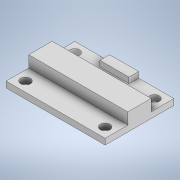
# Autodesk Inventor part: IMU-mpu6050
Saved by Autodesk Inventor 2022 (Build 260153000, 153)
## iProperties
Created: 2021-10-21
Part Number: IMU-mpu6050
Material: Generic
Document SubType Name: Modeling
Designer: kylem
Density: 1 g/cm^3
Appearance: Default
Author: kylem
Autodesk Inventor part; units mm, degrees
ref_plane "YZ Plane" through (0, 0, 0) normal (1, 0, 0) x (0, 1, 0)
ref_plane "XZ Plane" through (0, 0, 0) normal (0, 1, 0) x (-1, 0, 0)
sketch "Sketch1" plane through (0, 0, 0) normal (0, 1, 0) x (-1, 0, 0)
  line L0 (0, 0) -> (25.5, 0)
  line L1 (25.5, 0) -> (25.5, -17.7)
  line L2 (25.5, -17.7) -> (0, -17.7)
  line L3 (0, -17.7) -> (0, 0)
  dimension "d0" = 25.5
  dimension "d1" = 17.7
  constraints: 8 end point, 2 parallel, 1 horizontal, 1 perpendicular
  measures "d0" distance of L1.end L2.end
  measures "d1" distance of L0.end L1.end
extrude "Extrusion1" add sketch "Sketch1" along normal blind 1.54
sketch "Sketch2" plane through (0, 1.54, 0) normal (0, 1, 0) x (1, 0, 0)
  line L0 (-25.5, 0) -> (0, 0) projected
  line L1 (0, 0) -> (-2.5, 0)
  line L2 (-2.5, 0) -> (-2.5, 1.25)
  line L3 (-2.5, 2.5) -> (0, 2.5)
  line L4 (0, 2.5) -> (0, 0)
  circle A0 centre (-2.5, 2.5) radius 1.25
  line L5 (0, 17.7) -> (-25.5, 17.7) projected
  line L6 (0, 0) -> (0, 17.7)
  line L7 (0, 17.7) -> (0, 8.85)
  line L8 (0, 0) -> (0, 17.7) projected
  line L9 (0, 8.85) -> (-1.25, 8.85)
  line L10 (-25.5, 17.7) -> (0, 17.7)
  line L11 (-12.75, 17.7) -> (-12.75, 15.5963)
  circle A1 centre (-23, 2.5) radius 1.25
  circle A2 centre (-2.5, 15.2) radius 1.25
  circle A3 centre (-23, 15.2) radius 1.25
  dimension "d6" = 2.5
  dimension "d4" = 2.5
  dimension "d5" = 2.5
  constraints: 18 end point, 3 centre point, 3 symmetric about line, 2 horizontal, 2 midpoint, 2 parallel, 2 vertical, 1 coincident, 1 collinear, 1 perpendicular, 1 vertical alignment, 5 other
  measures "d4" distance of L3.start L3.end
  measures "d5" distance of L1.end L3.start
extrude "Extrusion2" cut sketch "Sketch2" against normal blind 1.54 contours A0 | A1 | A2 | A3
sketch "Sketch3" plane through (0, 0, 0) normal (1, 0, 0) x (0, 0, -1)
  line L0 (0, 0) -> (0, 1.54) projected
  line L1 (17.7, 0) -> (17.7, 1.54) projected
  line L2 (0, 0) -> (17.7, 0)
  line L3 (0, 0) -> (17.7, 0) projected
  line L4 (8.85, 0) -> (11.85, 0)
  line L5 (11.85, 0) -> (11.85, 4.5)
  line L6 (11.85, 4.5) -> (5.85, 4.5)
  line L7 (5.85, 4.5) -> (5.85, 0)
  line L8 (5.85, 4.5) -> (11.85, 4.5)
  line L9 (11.85, 4.5) -> (11.85, 0)
  line L10 (11.85, 0) -> (5.85, 0)
  line L11 (5.85, 0) -> (5.85, 4.5)
  dimension "d9" = 3
  dimension "d10" = 4.5
  dimension "d11" = 6
  constraints: 18 end point, 4 perpendicular, 2 horizontal, 2 parallel, 2 point on line, 1 midpoint
  measures "d9" distance of L4.start L4.end
  measures "d10" distance of L4.end L5.end
  measures "d11" distance of L5.end L6.end
extrude "Extrusion3" add sketch "Sketch3" against normal blind 25.5
sketch "Sketch4" plane through (0, 0, 0) normal (0, -1, 0) x (1, 0, 0)
  line L0 (0, -17.7) -> (-25.5, -17.7) projected
  line L1 (-9.0744, -17.7) -> (-16.5446, -17.7)
  line L2 (-16.5446, -17.7) -> (-16.5446, -15.2098)
  line L3 (-16.5446, -15.2098) -> (-9.0744, -15.2098)
  line L4 (-9.0744, -15.2098) -> (-9.0744, -17.7)
  point P0 (0, 0)
  constraints: 8 end point, 2 parallel, 1 horizontal, 1 perpendicular, 1 point on line
extrude "Extrusion4" add sketch "Sketch4" along normal blind 1.5
ref_plane "Work Plane1" through (0, 0.77, 0) normal (0, -1, 0) x (1, 0, 0)
mirror "Mirror1" about plane through (0, 0.77, 0) normal (0, -1, 0) of "Extrusion4"
body "Solid1"
